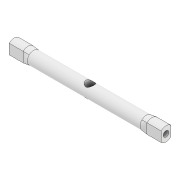
# Autodesk Inventor part: front shaft v2
Saved by Autodesk Inventor 2022 (Build 260153000, 153)
## iProperties
Created: 2024-03-20
Part Number: front shaft v2
Material: Generic
Document SubType Name: Modeling
Designer: david
Density: 1 g/cm^3
Appearance: Smooth - White
Author: david
Autodesk Inventor part; units mm, degrees
ref_plane "YZ Plane" through (0, 0, 0) normal (1, 0, 0) x (0, 1, 0)
sketch "Sketch1" plane through (0, 0, 0) normal (1, 0, 0) x (0, 1, 0)
  circle A0 centre (0, 0) radius 2.25
  dimension "diameter" = 4.5
  constraints: 1 centre point, 1 coincident
  measures "diameter" diameter of A0
extrude "Extrusion1" add sketch "Sketch1" along normal blind 20
ref_plane "Work Plane1" through (22, 0, 0) normal (1, 0, 0) x (0, 0, -1)
sketch "Sketch3" plane through (22, 0, 0) normal (1, 0, 0) x (0, 0, -1)
  arc A0 (-1.75, 1.7854) -> (-1.75, -1.7854) centre (0, 0) ccw construction
  line L0 (-1.75, -1.7854) -> (1.75, -1.7854) construction
  line L1 (1.75, -1.7854) -> (1.75, 1.7854)
  line L2 (1.75, 1.7854) -> (-1.75, 1.7854) construction
  line L3 (-1.75, 1.7854) -> (-1.75, -1.7854)
  line L4 (-1.75, -1.7854) -> (1.75, 1.7854) construction
  line L5 (1.75, -1.7854) -> (0, 0) construction
  arc A1 (1.75, 1.7854) -> (-1.75, 1.7854) centre (0, 0) ccw
  arc A2 (1.75, -1.7854) -> (1.75, 1.7854) centre (0, 0) ccw construction
  arc A3 (-1.75, -1.7854) -> (1.75, -1.7854) centre (0, 0) ccw
  line L6 (0, 0) -> (-1.75, 1.7854) construction
  dimension "d23" = 5
  dimension "d34" = 3.5
  constraints: 14 end point, 8 point on circle, 4 centre point, 2 parallel, 1 coincident, 1 horizontal, 1 midpoint, 1 perpendicular
  measures "d23" diameter of A0
  measures "d34" distance between parallel lines of L3 L1
extrude "Extrusion3" add sketch "Sketch3" along normal blind 5
loft "Loft1" add section 1 edges at (22, 2.5, 0) (22, 0, -1.75) (22, -2.5, 0) (22, 0, 1.75) section 2 edges at (20, -2.25, 0)
sketch "Sketch4" plane through (27, 0, 0) normal (1, 0, 0) x (0, 0, -1)
  arc A0 (1.75, 1.7854) -> (-1.75, 1.7854) centre (0, 0) ccw projected
  constraints: 1 coincident
hole "Hole1" at (27, 0, 0) direction (-1, 0, 0) diameter 2 depth 6
mirror "Mirror1" about plane through (0, 0, 0) normal (-1, 0, 0)
ref_plane "Work Plane2" through (0, 5, 0) normal (0, 1, 0) x (-1, 0, 0)
sketch "Sketch5" plane through (0, 5, 0) normal (0, 1, 0) x (-1, 0, 0)
  point P0 (0, 0)
  point P1 (0, 0)
  constraints: 1 coincident
hole "Hole2" at (0, 5, 0) direction (0, -1, 0) diameter 3 end through all counterbore diameter 6 counterbore depth 2
body "Solid1"
